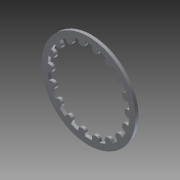
# Autodesk Inventor part: AT508
Saved by Autodesk Inventor 2014 (Build 180170000, 170)
## iProperties
Category: PARTsolutions
Company: NKKSWITCHES
Created: 2013-12-28
Part Number: AT508
Catalog Web Link: www.cadenas.de
Description: Lockwasher AT508 - Bushing Mount Miniature Toggles-Series M - Standard Hardwarw for Small & Large Bushings
Vendor: NKKSWITCHES
Document SubType Name: Modeling
Designer: PARTuser1
Manufacturer: NKKSWITCHES
Density: 1 g/cm^3
Material: Generic
Appearance: RGB(192.00000375509219,192.00000375509219,192.00000375509219)
PSOL_IDENT_0: {$CADENAS_DATA\23d-libs\nkkswitches\toggle\m\hardware\lockwasher_at508.prj},187 {VTYP=3D},{NB=AT508}
PSOL_IDENT_1: ,{LINA=AT508},{NN=Lockwasher AT508 - Bushing Mount Miniature Toggles},{DATE=16.01.2007 11:58:47},{GE
PSOL_IDENT_2: OMDATE=11.10.2006},{VERSION=},{LINEID=10},{LINESUBID=-1},{WBVAR=}  {NB=AT508},{LINA=AT508},{KT=DUMMY
PSOL_IDENT_3: },{PN=AT508},{D=0.622},{DD=0.476},{T=0.020},{D3=0.543}
CNS_NN: Lockwasher AT508 - Bushing Mount Miniature Toggles
CNS_NT: Series M - Standard Hardwarw for Small & Large Bushings
CNS_NB: AT508
CNS_NBSYN: $PN.
CNS_LINA: AT508
CNS_PN: AT508
CNS_D: 0.622
CNS_DD: 0.476
CNS_T: 0.020
CNS_D3: 0.543
SUPPLIER: NKKSWITCHES
ARTICLENO: AT508
BOMINFO: AT508
CREATOR: CADENAS GmbH
Title: AT508
Author: Cadenas PARTsolutions
Comments: Series M - Standard Hardwarw for Small & Large Bushings
Autodesk Inventor part; units mm, degrees
sketch "Sketch_2" plane through (0, 0, 0) normal (0, 0, 1) x (1, 0, 0)
  circle A0 centre (0, 0) radius 7.8994
  line L0 (-6.8699, 0.601) -> (-6.5086, 0.5694)
  arc A1 (-6.0489, 0) -> (-6.5086, 0.5694) centre (-6.5529, 0.0634) ccw
  arc A2 (-6.5086, -0.5694) -> (-6.0489, 0) centre (-6.5529, -0.0634) ccw
  line L1 (-6.5086, -0.5694) -> (-6.8699, -0.601)
  arc A3 (-6.8699, -0.601) -> (-6.6611, -1.7848) centre (0, 0) ccw
  line L2 (-6.6611, -1.7848) -> (-6.3109, -1.691)
  arc A4 (-5.6841, -2.0688) -> (-6.3109, -1.691) centre (-6.1794, -2.1817) ccw
  arc A5 (-5.9213, -2.7612) -> (-5.6841, -2.0688) centre (-6.136, -2.3008) ccw
  line L3 (-5.9213, -2.7612) -> (-6.25, -2.9144)
  arc A6 (-6.25, -2.9144) -> (-5.649, -3.9554) centre (0, 0) ccw
  line L4 (-5.649, -3.9554) -> (-5.3519, -3.7475)
  arc A7 (-4.6337, -3.8881) -> (-5.3519, -3.7475) centre (-5.0605, -4.1636) ccw
  arc A8 (-4.6199, -4.6199) -> (-4.6337, -3.8881) centre (-4.9791, -4.2607) ccw
  line L5 (-4.6199, -4.6199) -> (-4.8763, -4.8763)
  arc A9 (-4.8763, -4.8763) -> (-3.9554, -5.649) centre (0, 0) ccw
  line L6 (-3.9554, -5.649) -> (-3.7475, -5.3519)
  arc A10 (-3.0244, -5.2385) -> (-3.7475, -5.3519) centre (-3.3313, -5.6433) ccw
  arc A11 (-2.7612, -5.9213) -> (-3.0244, -5.2385) centre (-3.2216, -5.7067) ccw
  line L7 (-2.7612, -5.9213) -> (-2.9144, -6.25)
  arc A12 (-2.9144, -6.25) -> (-1.7848, -6.6611) centre (0, 0) ccw
  line L8 (-1.7848, -6.6611) -> (-1.691, -6.3109)
  arc A13 (-1.0504, -5.957) -> (-1.691, -6.3109) centre (-1.2003, -6.4423) ccw
  arc A14 (-0.5694, -6.5086) -> (-1.0504, -5.957) centre (-1.0755, -6.4643) ccw
  line L9 (-0.5694, -6.5086) -> (-0.601, -6.8699)
  arc A15 (-0.601, -6.8699) -> (0.601, -6.8699) centre (0, 0) ccw
  line L10 (0.601, -6.8699) -> (0.5694, -6.5086)
  arc A16 (1.0504, -5.957) -> (0.5694, -6.5086) centre (1.0755, -6.4643) ccw
  arc A17 (1.691, -6.3109) -> (1.0504, -5.957) centre (1.2003, -6.4423) ccw
  line L11 (1.691, -6.3109) -> (1.7848, -6.6611)
  arc A18 (1.7848, -6.6611) -> (2.9144, -6.25) centre (0, 0) ccw
  line L12 (2.9144, -6.25) -> (2.7612, -5.9213)
  arc A19 (3.0244, -5.2385) -> (2.7612, -5.9213) centre (3.2216, -5.7067) ccw
  arc A20 (3.7475, -5.3519) -> (3.0244, -5.2385) centre (3.3313, -5.6433) ccw
  line L13 (3.7475, -5.3519) -> (3.9554, -5.649)
  arc A21 (3.9554, -5.649) -> (4.8763, -4.8763) centre (0, 0) ccw
  line L14 (4.8763, -4.8763) -> (4.6199, -4.6199)
  arc A22 (4.6337, -3.8881) -> (4.6199, -4.6199) centre (4.9791, -4.2607) ccw
  arc A23 (5.3519, -3.7475) -> (4.6337, -3.8881) centre (5.0605, -4.1636) ccw
  line L15 (5.3519, -3.7475) -> (5.649, -3.9554)
  arc A24 (5.649, -3.9554) -> (6.25, -2.9144) centre (0, 0) ccw
  line L16 (6.25, -2.9144) -> (5.9213, -2.7612)
  arc A25 (5.6841, -2.0688) -> (5.9213, -2.7612) centre (6.136, -2.3008) ccw
  arc A26 (6.3109, -1.691) -> (5.6841, -2.0688) centre (6.1794, -2.1817) ccw
  line L17 (6.3109, -1.691) -> (6.6611, -1.7848)
  arc A27 (6.6611, -1.7848) -> (6.8699, -0.601) centre (0, 0) ccw
  line L18 (6.8699, -0.601) -> (6.5086, -0.5694)
  arc A28 (6.0489, 0) -> (6.5086, -0.5694) centre (6.5529, -0.0634) ccw
  arc A29 (6.5086, 0.5694) -> (6.0489, 0) centre (6.5529, 0.0634) ccw
  line L19 (6.5086, 0.5694) -> (6.8699, 0.601)
  arc A30 (6.8699, 0.601) -> (6.6611, 1.7848) centre (0, 0) ccw
  line L20 (6.6611, 1.7848) -> (6.3109, 1.691)
  arc A31 (5.6841, 2.0688) -> (6.3109, 1.691) centre (6.1794, 2.1817) ccw
  arc A32 (5.9213, 2.7612) -> (5.6841, 2.0688) centre (6.136, 2.3008) ccw
  line L21 (5.9213, 2.7612) -> (6.25, 2.9144)
  arc A33 (6.25, 2.9144) -> (5.649, 3.9554) centre (0, 0) ccw
  line L22 (5.649, 3.9554) -> (5.3519, 3.7475)
  arc A34 (4.6337, 3.8881) -> (5.3519, 3.7475) centre (5.0605, 4.1636) ccw
  arc A35 (4.6199, 4.6199) -> (4.6337, 3.8881) centre (4.9791, 4.2607) ccw
  line L23 (4.6199, 4.6199) -> (4.8763, 4.8763)
  arc A36 (4.8763, 4.8763) -> (3.9554, 5.649) centre (0, 0) ccw
  line L24 (3.9554, 5.649) -> (3.7475, 5.3519)
  arc A37 (3.0244, 5.2385) -> (3.7475, 5.3519) centre (3.3313, 5.6433) ccw
  arc A38 (2.7612, 5.9213) -> (3.0244, 5.2385) centre (3.2216, 5.7067) ccw
  line L25 (2.7612, 5.9213) -> (2.9144, 6.25)
  arc A39 (2.9144, 6.25) -> (1.7848, 6.6611) centre (0, 0) ccw
  line L26 (1.7848, 6.6611) -> (1.691, 6.3109)
  arc A40 (1.0504, 5.957) -> (1.691, 6.3109) centre (1.2003, 6.4423) ccw
  arc A41 (0.5694, 6.5086) -> (1.0504, 5.957) centre (1.0755, 6.4643) ccw
  line L27 (0.5694, 6.5086) -> (0.601, 6.8699)
  arc A42 (0.601, 6.8699) -> (-0.601, 6.8699) centre (0, 0) ccw
  line L28 (-0.601, 6.8699) -> (-0.5694, 6.5086)
  arc A43 (-1.0504, 5.957) -> (-0.5694, 6.5086) centre (-1.0755, 6.4643) ccw
  arc A44 (-1.691, 6.3109) -> (-1.0504, 5.957) centre (-1.2003, 6.4423) ccw
  line L29 (-1.691, 6.3109) -> (-1.7848, 6.6611)
  arc A45 (-1.7848, 6.6611) -> (-2.9144, 6.25) centre (0, 0) ccw
  line L30 (-2.9144, 6.25) -> (-2.7612, 5.9213)
  arc A46 (-3.0244, 5.2385) -> (-2.7612, 5.9213) centre (-3.2216, 5.7067) ccw
  arc A47 (-3.7475, 5.3519) -> (-3.0244, 5.2385) centre (-3.3313, 5.6433) ccw
  line L31 (-3.7475, 5.3519) -> (-3.9554, 5.649)
  arc A48 (-3.9554, 5.649) -> (-4.8763, 4.8763) centre (0, 0) ccw
  line L32 (-4.8763, 4.8763) -> (-4.6199, 4.6199)
  arc A49 (-4.6337, 3.8881) -> (-4.6199, 4.6199) centre (-4.9791, 4.2607) ccw
  arc A50 (-5.3519, 3.7475) -> (-4.6337, 3.8881) centre (-5.0605, 4.1636) ccw
  line L33 (-5.3519, 3.7475) -> (-5.649, 3.9554)
  arc A51 (-5.649, 3.9554) -> (-6.25, 2.9144) centre (0, 0) ccw
  line L34 (-6.25, 2.9144) -> (-5.9213, 2.7612)
  arc A52 (-5.6841, 2.0688) -> (-5.9213, 2.7612) centre (-6.136, 2.3008) ccw
  arc A53 (-6.3109, 1.691) -> (-5.6841, 2.0688) centre (-6.1794, 2.1817) ccw
  line L35 (-6.3109, 1.691) -> (-6.6611, 1.7848)
  arc A54 (-6.6611, 1.7848) -> (-6.8699, 0.601) centre (0, 0) ccw
  constraints: 108 point on circle, 72 end point, 55 centre point
extrude "Extrusion1" add sketch "Sketch_2" along normal mid plane 0.508
ref_plane "lockwasher_XY" through (0, 0, 0.254) normal (0, 0, 1) x (1, 0, 0)
ref_plane "lockwasher_YZ" through (0, 0, 0.254) normal (1, 0, 0) x (0, 1, 0)
ref_plane "lockwasher_ZX" through (0, 0, 0.254) normal (0, 1, 0) x (0, 0, 1)
body "Solid1"
